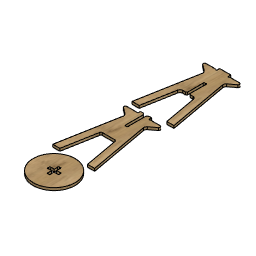
week08_cnc_bench (Autodesk Fusion 360 design; units mm, degrees)
Autodesk Fusion 360 part; units mm, degrees
sketch "Sketch1" plane through (0, 0, 0) normal (0, 1, 0) x (1, 0, 0)
  line L0 (300, 0) -> (300, 500) construction
  line L1 (0, 500) -> (0, 0) construction
  line L2 (0, 0) -> (77.7889, 427.8387)
  line L3 (70.1115, 447.4164) -> (24, 482)
  line L4 (300, 0) -> (222.2111, 427.8387)
  line L5 (229.8885, 447.4164) -> (276, 482)
  line L6 (0, 0) -> (50.8197, 0)
  line L7 (249.1803, 0) -> (300, 0)
  line L8 (141.25, 375) -> (141.25, 257.0711)
  line L9 (159.25, 375) -> (159.25, 257.0711)
  line L10 (112.9658, 250) -> (134.1789, 250)
  line L11 (166.321, 250) -> (187.0342, 250)
  line L12 (141.25, 375) -> (159.25, 375)
  line L13 (206.7116, 233.5777) -> (225.8048, 128.565)
  line L14 (234.8957, 78.565) -> (249.1803, 0)
  line L15 (50.8197, 0) -> (65.1043, 78.565)
  line L16 (74.1952, 128.565) -> (93.2884, 233.5777)
  line L17 (234.8957, 78.565) -> (225.8048, 128.565)
  line L18 (74.1952, 128.565) -> (65.1043, 78.565)
  arc A0 (30, 500) -> (24, 482) centre (30, 490) ccw
  arc A1 (276, 482) -> (270, 500) centre (270, 490) ccw
  arc A2 (77.7889, 427.8387) -> (70.1115, 447.4164) centre (58.1115, 431.4164) ccw
  arc A3 (229.8885, 447.4164) -> (222.2111, 427.8387) centre (241.8885, 431.4164) ccw
  arc A4 (206.7116, 233.5777) -> (187.0342, 250) centre (187.0342, 230) ccw
  arc A5 (112.9658, 250) -> (93.2884, 233.5777) centre (112.9658, 230) ccw
  line L19 (134.1789, 250) -> (141.25, 257.0711)
  line L20 (166.321, 250) -> (159.25, 257.0711)
  line L21 (110, 510) -> (110, 517.5)
  line L22 (110, 517.5) -> (190, 517.5)
  line L23 (190, 517.5) -> (190, 510)
  line L24 (270, 500) -> (200, 500)
  line L25 (100, 500) -> (30, 500)
  line L26 (110, 510) -> (110, 500)
  arc A6 (100, 500) -> (110, 500) centre (105, 500) ccw
  line L27 (190, 510) -> (190, 500)
  arc A7 (190, 500) -> (200, 500) centre (195, 500) ccw
  point P0 (80, 440)
  point P1 (159.25, 250)
  point P2 (141.25, 250)
  dimension "d1" = 300
  dimension "d3" = 500
  dimension "d4" = 80
  dimension "d5" = 60
  dimension "d6" = 18
  dimension "d7" = 125
  dimension "d10" = 250
  dimension "d11" = 50
  dimension "d29" = 10
  dimension "d30" = 20
  dimension "d31" = 7.071
  dimension "d32" = 7.071
  dimension "d33" = 7.071
  dimension "d34" = 7.071
  dimension "d39" = 17.5
  dimension "d132" = 10
  constraint vertical L0
  constraint horizontal L24
  constraint vertical L1
  constraint coincident L1.end L2.start
  constraint parallel L2 L15
  constraint parallel L4 L13
  constraint horizontal L10
  constraint perpendicular L8 L10
  constraint coincident P1 L10
  constraint perpendicular L9 L10
  constraint collinear L10 L11
  constraint perpendicular L9 L12
  constraint equal L6 L7
  constraint collinear L6 L7
  constraint coincident L14.start L13
  constraint collinear L13 L14
  constraint collinear L15 L16
  constraint coincident L16.start L15
  constraint coincident L1.start L3
  constraint coincident L1.start L24
  constraint tangent L3 A0
  constraint tangent A0 L24
  constraint coincident L0.end L5
  constraint coincident L0.end L24
  constraint tangent L5 A1
  constraint tangent A1 L24
  constraint equal A0 A1
  constraint coincident P0 L2
  constraint coincident P0 L3
  constraint tangent L2 A2
  constraint tangent L3 A2
  constraint tangent L4 A3
  constraint tangent L5 A3
  constraint equal A2 A3
  constraint tangent L13 A4
  constraint tangent L11 A4
  constraint equal A2 A4
  constraint tangent L10 A5
  constraint tangent L16 A5
  constraint equal A2 A5
  constraint coincident L10 P2
  constraint coincident L8 P2
  constraint coincident P1 L9
  constraint vertical L21
  constraint horizontal L22
  constraint vertical L23
  constraint collinear L24 L25
  constraint coincident L27.end L24
  constraint coincident L27.end L23
  constraint tangent L26 A6
  constraint coincident L27.end A7.start
  measures "d1" distance of L0.end L1.start
  measures "d3" distance of L0.start L0.end
  measures "d4" distance of L1 P0
  measures "d5" distance of P0 L24
  measures "d6" distance of L8.start L9.start
  measures "d7" distance of L9.start P1
  measures "d10" distance of P1 L24
  measures "d11" distance of L2 L15
  measures "d29" radius of A0
  measures "d30" radius of A2
  measures "d31" distance of L10.end P2
  measures "d32" distance of L8.end P2
  measures "d33" distance of P1 L11.start
  measures "d34" distance of P1 L9.end
  measures "d39" distance of L27.end L22.end
  measures "d132" diameter of A7
extrude "Extrude1" add sketch "Sketch1" along normal blind 18 makes body 1
sketch "Sketch2" plane through (0, 0, 0) normal (0, 1, 0) x (1, 0, 0)
  line L0 (0, 0) -> (77.7889, 427.8387)
  line L1 (74.1952, 128.565) -> (94.7813, 241.7889)
  line L2 (70.1115, 447.4164) -> (24, 482)
  line L3 (104.62, 250) -> (141.25, 250)
  line L4 (159.25, 250) -> (195.38, 250)
  line L5 (300, 0) -> (300, 500) construction
  line L6 (50.8197, 0) -> (65.1043, 78.565)
  line L7 (205.2187, 241.7889) -> (225.8048, 128.565)
  line L8 (229.8885, 447.4164) -> (276, 482)
  line L9 (234.8957, 78.565) -> (249.1803, 0)
  line L10 (300, 0) -> (222.2111, 427.8387)
  line L11 (0, 500) -> (0, 0) construction
  line L12 (0, 0) -> (50.8197, 0)
  line L13 (249.1803, 0) -> (300, 0)
  line L14 (159.25, 375) -> (141.25, 375)
  line L15 (141.25, 375) -> (141.25, 508)
  line L16 (159.25, 508) -> (159.25, 375)
  line L17 (141.25, 250) -> (159.25, 250)
  line L18 (270, 500) -> (190, 500)
  line L19 (110, 500) -> (30, 500)
  line L20 (65.1043, 78.565) -> (74.1952, 128.565)
  line L21 (225.8048, 128.565) -> (234.8957, 78.565)
  arc A0 (229.8885, 447.4164) -> (222.2111, 427.8387) centre (241.8885, 431.4164) ccw
  arc A1 (77.7889, 427.8387) -> (70.1115, 447.4164) centre (58.1115, 431.4164) ccw
  arc A2 (205.2187, 241.7889) -> (195.38, 250) centre (195.38, 240) ccw
  arc A3 (104.62, 250) -> (94.7813, 241.7889) centre (104.62, 240) ccw
  arc A4 (30, 500) -> (24, 482) centre (30, 490) ccw
  arc A5 (276, 482) -> (270, 500) centre (270, 490) ccw
  line L22 (141.25, 500) -> (159.25, 500)
  line L23 (190, 500) -> (190, 518)
  line L24 (110, 518) -> (110, 500)
  line L25 (190, 518) -> (169.25, 518)
  line L26 (131.25, 518) -> (110, 518)
  line L27 (141.25, 508) -> (131.25, 518)
  line L28 (159.25, 508) -> (169.25, 518)
  point P0 (80, 440)
  point P1 (141.25, 518)
  point P2 (159.25, 518)
  dimension "d14" = 300
  dimension "d15" = 500
  dimension "d16" = 80
  dimension "d17" = 60
  dimension "d19" = 125
  dimension "d20" = 250
  dimension "d21" = 50
  dimension "d26" = 18
  dimension "d27" = 20
  dimension "d28" = 10
  dimension "d41" = 18
  dimension "d42" = 10
  dimension "d43" = 10
  dimension "d44" = 10
  dimension "d45" = 10
  constraint vertical L5
  constraint horizontal L18
  constraint vertical L11
  constraint coincident L0.start L11.end
  constraint parallel L0 L6
  constraint parallel L7 L10
  constraint horizontal L3
  constraint coincident L4.start L3
  constraint collinear L3 L4
  constraint equal L12 L13
  constraint collinear L12 L13
  constraint coincident L9.start L7
  constraint collinear L7 L9
  constraint collinear L1 L6
  constraint coincident L1.start L6
  constraint horizontal L14
  constraint vertical L15
  constraint vertical L16
  constraint collinear L18 L19
  constraint tangent L10 A0
  constraint tangent L8 A0
  constraint coincident P0 L0
  constraint coincident P0 L2
  constraint tangent L0 A1
  constraint tangent L2 A1
  constraint equal A0 A1
  constraint tangent L7 A2
  constraint tangent L4 A2
  constraint tangent L1 A3
  constraint tangent L3 A3
  constraint equal A2 A3
  constraint coincident L11.start L2
  constraint coincident L11.start L19
  constraint tangent L2 A4
  constraint tangent L19 A4
  constraint equal A2 A4
  constraint coincident L5.end L8
  constraint coincident L5.end L18
  constraint tangent L8 A5
  constraint tangent L18 A5
  constraint equal A2 A5
  constraint horizontal L22
  constraint vertical L23
  constraint horizontal L25
  constraint vertical L24
  constraint coincident L15 L22.start
  constraint coincident L16 L22.end
  constraint collinear L25 L26
  constraint coincident L15 P1
  constraint coincident L26 P1
  constraint coincident L16 P2
  constraint coincident L25 P2
  constraint equal L18 L19
  measures "d14" distance of L11.start L5.end
  measures "d15" distance of L5.start L5.end
  measures "d16" distance of P0 L11
  measures "d17" distance of P0 L18
  measures "d19" distance of L4.start L14.start
  measures "d20" distance of L4.start L18
  measures "d21" distance of L0 L6
  measures "d26" distance of L15 L16
  measures "d27" radius of A0
  measures "d28" radius of A2
  measures "d41" distance of L19.start L24.start
  measures "d42" distance of L15.end P1
  measures "d43" distance of L26.start P1
  measures "d44" distance of L16.start P2
  measures "d45" distance of L25.end P2
extrude "Extrude2" add sketch "Sketch2" along normal blind 18 separate body contours L0 L1 L2 L3 L4 L6 L7 L8 L9 L10 L12 L13 L14 L15 L16 L17 L18 L19 L20 L21 A0 A1 A2 A3 A4 A5 L23 L24 L25 L26 L27 L28 makes body 2
move_body "Move1" bodies 2 to x (1, 0, 0) y (0, 1, 0) z (0, 0, 1) at (0, 0, 0)
move_body "Move2" bodies 2 to x (1, 0, 0) y (0, 1, 0) z (0, 0, 1) at (-18, 0, 0)
sketch "Sketch3" plane through (0, 0, 0) normal (0, 1, 0) x (1, 0, 0)
  circle A0 centre (-150.954, 11.058) radius 150
  line L0 (-190.9093, 52) -> (-110.9988, 52) construction
  line L1 (-110.9988, 52) -> (-110.9988, -29.8839) construction
  line L2 (-110.9988, -29.8839) -> (-190.9093, -29.8839) construction
  line L3 (-190.9093, -29.8839) -> (-190.9093, 52) construction
  line L4 (-190.9093, 52) -> (-110.9988, -29.8839) construction
  line L5 (-110.9988, 52) -> (-190.9093, -29.8839) construction
  line L6 (-159.954, 52) -> (-141.954, 52)
  line L7 (-141.954, -29.8839) -> (-159.954, -29.8839)
  line L8 (-159.954, 52) -> (-141.954, -29.8839) construction
  line L9 (-141.954, 52) -> (-159.954, -29.8839) construction
  line L10 (-110.9988, 20.058) -> (-110.9988, 2.058)
  line L11 (-190.9093, 2.058) -> (-190.9093, 20.058)
  line L12 (-190.9093, 20.058) -> (-110.9988, 2.058) construction
  line L13 (-110.9988, 20.058) -> (-190.9093, 2.058) construction
  line L14 (-190.9093, 20.058) -> (-159.954, 20.058)
  line L15 (-159.954, 20.058) -> (-159.954, 52)
  line L16 (-141.954, 52) -> (-141.954, 20.058)
  line L17 (-141.954, 20.058) -> (-110.9988, 20.058)
  line L18 (-141.954, 2.058) -> (-141.954, -29.8839)
  line L19 (-110.9988, 2.058) -> (-141.954, 2.058)
  line L20 (-159.954, 2.058) -> (-190.9093, 2.058)
  line L21 (-159.954, -29.8839) -> (-159.954, 2.058)
  point P0 (-150.954, 11.058)
  point P1 (-150.954, 11.058)
  point P2 (-150.954, 11.058)
  dimension "d46" = 300
  dimension "d55" = 18
  dimension "d56" = 18
  constraint horizontal L0
  constraint perpendicular L0 L1
  constraint parallel L0 L2
  constraint parallel L1 L3
  constraint coincident L4 P2
  constraint coincident L5 P2
  constraint coincident P2 P0
  constraint horizontal L6
  constraint perpendicular L6 L16
  constraint parallel L6 L7
  constraint parallel L16 L21
  constraint coincident L0 L6.start
  constraint coincident L8 P2
  constraint coincident L9 P2
  constraint coincident P2 P1
  constraint horizontal L14
  constraint perpendicular L10 L14
  constraint parallel L14 L19
  constraint parallel L10 L11
  constraint coincident L3 L11.end
  constraint coincident L12 P2
  constraint coincident L13 P2
  constraint coincident L14.end L21
  constraint collinear L15 L21
  measures "d46" diameter of A0
  measures "d55" distance of L14 L19
  measures "d56" distance of L6.start L6.end
extrude "Extrude3" add sketch "Sketch3" along normal blind 18 separate body makes body 3
move_body "Move3" bodies 3 to x (1, 0, 0) y (0, 1, 0) z (0, 0, 1) at (0, -1.25, 18.5)
move_body "Move13" bodies 1 to x (1, 0, 0) y (0, 1, 0) z (0, 0, 1) at (0, 0, -550)
move_body "Move14" bodies 3 to x (1, 0, 0) y (0, 1, 0) z (0, 0, 1) at (300, 0, 150)
hole "Hole1" at (154.5104, -1.25, 194.8484) direction (0, 1, 0) diameter 10 end up to surface (18 mm away) bodies 3
hole "Hole2" at (185.4657, -1.25, 162.9064) direction (0, 1, 0) diameter 10 end up to surface (18 mm away) bodies 3
hole "Hole3" at (185.4657, -1.25, 151.9775) direction (0, 1, 0) diameter 10 end up to surface (18 mm away) bodies 3
hole "Hole4" at (154.5104, -1.25, 120.0355) direction (0, 1, 0) diameter 10 end up to surface (18 mm away) bodies 3
hole "Hole5" at (143.5815, -1.25, 120.0355) direction (0, 1, 0) diameter 10 end up to surface (18 mm away) bodies 3
hole "Hole6" at (112.6262, -1.25, 151.9775) direction (0, 1, 0) diameter 10 end up to surface (18 mm away) bodies 3
hole "Hole7" at (112.6262, -1.25, 162.9064) direction (0, 1, 0) diameter 10 end up to surface (18 mm away) bodies 3
hole "Hole8" at (143.5815, -1.25, 194.8484) direction (0, 1, 0) diameter 10 end up to surface (18 mm away) bodies 3
hole "Hole9" at (137.7145, 0, -378.5355) direction (0, 1, 0) diameter 10 end up to surface (18 mm away) bodies 2
hole "Hole10" at (175.5355, 0, -503.5355) direction (0, 1, 0) diameter 10 end up to surface (18 mm away) bodies 2
hole "Hole11" at (88.4645, 0, -503.5355) direction (0, 1, 0) diameter 10 end up to surface (18 mm away) bodies 2
hole "Hole12" at (126.7855, 0, -378.5355) direction (0, 1, 0) diameter 10 end up to surface (18 mm away) bodies 2
hole "Hole13" at (155.7145, 0, -921.4645) direction (0, 1, 0) diameter 10 end up to surface (18 mm away) bodies 1
hole "Hole14" at (144.7855, 0, -921.4645) direction (0, 1, 0) diameter 10 end up to surface (18 mm away) bodies 1
equation "d8 = d6"
equation "d14 = d1"
equation "d15 = d3"
equation "d16 = d4"
equation "d17 = d5"
equation "d19 = d10 / 2"
equation "d20 = d10"
equation "d21 = d11"
equation "d24 = d6"
equation "d26 = d6"
equation "d32 = d31"
equation "d34 = d33"
equation "d41 = d6"
equation "d43 = d42"
equation "d45 = d44"
equation "d53 = d6"
equation "d55 = d6"
equation "d56 = d6"
equation "dbToolDia = 10 mm"
equation "dbOffset = 0 mm" comment "Do NOT change formula"
equation "dbRadius = ( dbToolDia + dbOffset ) / 2" comment "Do NOT change formula"
equation "dbMinPercent = 10"
equation "dbHoleOffset = dbRadius / sqrt(2)" comment "Do NOT change formula"
equation "HoleDepth = 10.00 mm"
equation "HoleDiameter = dbRadius * 2"
equation "TipAngle = 180 deg"
equation "RefDim1 = dbHoleOffset"
equation "RefDim2 = dbHoleOffset"
equation "d68 = dbRadius * 2"
equation "d70 = dbHoleOffset"
equation "d71 = dbHoleOffset"
equation "d73 = dbRadius * 2"
equation "d75 = dbHoleOffset"
equation "d76 = dbHoleOffset"
equation "d78 = dbRadius * 2"
equation "d80 = dbHoleOffset"
equation "d81 = dbHoleOffset"
equation "d83 = dbRadius * 2"
equation "d85 = dbHoleOffset"
equation "d86 = dbHoleOffset"
equation "d88 = dbRadius * 2"
equation "d90 = dbHoleOffset"
equation "d91 = dbHoleOffset"
equation "d93 = dbRadius * 2"
equation "d95 = dbHoleOffset"
equation "d96 = dbHoleOffset"
equation "d98 = dbRadius * 2"
equation "d100 = dbHoleOffset"
equation "d101 = dbHoleOffset"
equation "d103 = dbRadius * 2"
equation "d105 = dbHoleOffset"
equation "d106 = dbHoleOffset"
equation "d108 = dbRadius * 2"
equation "d110 = dbHoleOffset"
equation "d111 = dbHoleOffset"
equation "d113 = dbRadius * 2"
equation "d115 = dbHoleOffset"
equation "d116 = dbHoleOffset"
equation "d118 = dbRadius * 2"
equation "d120 = dbHoleOffset"
equation "d121 = dbHoleOffset"
equation "d123 = dbRadius * 2"
equation "d125 = dbHoleOffset"
equation "d126 = dbHoleOffset"
equation "d128 = dbRadius * 2"
equation "d130 = dbHoleOffset"
equation "d131 = dbHoleOffset"
